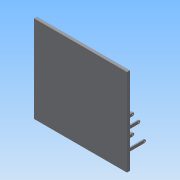
# Autodesk Inventor part: 0
Saved by Autodesk Inventor 2015 (Build 190159000, 159)
## iProperties
Created: 2018-05-07
Part Number: 0
Material: 一般
Document SubType Name: Modeling
Designer: 王博聖
Density: 1 g/cm^3
Appearance: 預設
Author: 王博聖
Autodesk Inventor part; units mm, degrees
ref_plane "YZ Plane" through (0, 0, 0) normal (1, 0, 0) x (0, 1, 0)
ref_plane "XZ Plane" through (0, 0, 0) normal (0, 1, 0) x (-1, 0, 0)
sketch "草圖1" plane through (0, 0, 0) normal (0, 1, 0) x (-1, 0, 0)
  line L0 (0, 0) -> (160, 0)
  line L1 (160, 0) -> (160, -130)
  line L2 (160, -130) -> (0, -130)
  line L3 (0, -130) -> (0, 0)
  dimension "d0" = 160
  dimension "d1" = 130
  constraints: 8 end point, 2 parallel, 1 horizontal, 1 perpendicular
  measures "d0" distance of L1.end L2.end
  measures "d1" distance of L0.end L1.end
extrude "擠出1" add sketch "草圖1" along normal blind 5
sketch "草圖2" plane through (0, 0, 0) normal (1, 0, 0) x (0, 0, -1)
  line L0 (130, 0) -> (0, 0) projected
  line L1 (65, 0) -> (65, 20.4)
  line L2 (65, 20.4) -> (65, 0) construction
  line L3 (62.5, 20.4) -> (62.5, 0)
  line L4 (67.5, 0) -> (67.5, 20.4)
  arc A0 (67.5, 20.4) -> (62.5, 20.4) centre (65, 20.4) ccw
  arc A1 (62.5, 0) -> (67.5, 0) centre (65, 0) ccw construction
  line L5 (67.5, 0) -> (62.5, 0)
  circle A2 centre (65, 20.4) radius 1.25
  point P0 (65, 10.2)
  dimension "d4" = 20.4
  dimension "d5" = 5
  dimension "d6" = 2.5
  constraints: 12 end point, 4 point on circle, 4 tangent, 3 centre point, 2 collinear, 2 midpoint, 1 coincident, 1 parallel, 1 vertical
  measures "d4" distance of L1.start L1.end
  measures "d5" diameter of A1
  measures "d6" diameter of A2
extrude "擠出2" add sketch "草圖2" against normal blind 2
sketch "草圖3" plane through (0, 0, 0) normal (1, 0, 0) x (0, 0, -1)
  line L0 (130, 0) -> (0, 0) construction
  arc A0 (67.5, 20.4) -> (62.5, 20.4) centre (65, 20.4) ccw projected
  line L1 (65, 20.4) -> (48.2, 20.4) construction
  line L2 (48.2, 20.4) -> (48.2, 10) construction
  line L3 (48.2, 10) -> (48.2, 0) construction
  line L4 (45.7, 10) -> (45.7, 0)
  line L5 (50.7, 0) -> (50.7, 10)
  arc A1 (50.7, 10) -> (45.7, 10) centre (48.2, 10) ccw
  arc A2 (45.7, 0) -> (50.7, 0) centre (48.2, 0) ccw construction
  circle A3 centre (48.2, 10) radius 1.25
  line L6 (50.7, 0) -> (45.7, 0)
  line L7 (65, 20.4) -> (42, 20.4) construction
  line L8 (42, 20.4) -> (42, 10) construction
  line L9 (42, 10) -> (42, 0) construction
  line L10 (39.5, 10) -> (39.5, 0)
  line L11 (44.5, 0) -> (44.5, 10)
  arc A4 (44.5, 10) -> (39.5, 10) centre (42, 10) ccw
  arc A5 (39.5, 0) -> (44.5, 0) centre (42, 0) ccw construction
  circle A6 centre (42, 10) radius 1.25
  line L12 (44.5, 0) -> (39.5, 0)
  circle A7 centre (65, 20.4) radius 1.25 projected
  line L13 (65, 20.4) -> (78.6, 20.4) construction
  line L14 (78.6, 20.4) -> (78.6, 10) construction
  line L15 (78.6, 10) -> (78.6, 0) construction
  line L16 (76.1, 10) -> (76.1, 0)
  line L17 (81.1, 0) -> (81.1, 10)
  arc A8 (81.1, 10) -> (76.1, 10) centre (78.6, 10) ccw
  arc A9 (76.1, 0) -> (81.1, 0) centre (78.6, 0) ccw construction
  circle A10 centre (78.6, 10) radius 1.25
  line L18 (81.1, 0) -> (76.1, 0)
  line L19 (81.1, 0) -> (76.1, 0)
  line L20 (0, 0) -> (130, 0) projected
  line L21 (65, 20.4) -> (65, 30.17) construction
  line L22 (65, 30.17) -> (98.58, 30.17) construction
  line L23 (98.58, 30.17) -> (98.58, 0) construction
  line L24 (96.08, 30.17) -> (96.08, 0)
  line L25 (101.08, 0) -> (101.08, 30.17)
  arc A11 (101.08, 30.17) -> (96.08, 30.17) centre (98.58, 30.17) ccw
  arc A12 (96.08, 0) -> (101.08, 0) centre (98.58, 0) ccw construction
  circle A13 centre (98.58, 30.17) radius 1.25
  line L26 (101.08, 0) -> (96.08, 0)
  point P0 (48.2, 5)
  point P1 (42, 5)
  point P2 (78.6, 5)
  point P3 (98.58, 15.085)
  dimension "d9" = 16.8
  dimension "d11" = 10.4
  dimension "d12" = 5
  dimension "d13" = 2.5
  dimension "d14" = 23
  dimension "d15" = 10.4
  dimension "d16" = 5
  dimension "d17" = 2.5
  dimension "d20" = 13.6
  dimension "d21" = 10.4
  dimension "d22" = 5
  dimension "d23" = 2.5
  dimension "d24" = 9.77
  dimension "d25" = 33.58
  dimension "d26" = 5
  dimension "d27" = 2.5
  constraints: 58 end point, 16 point on circle, 16 tangent, 12 centre point, 8 perpendicular, 4 coincident, 4 horizontal, 4 midpoint, 4 parallel, 4 point on line, 3 collinear, 2 vertical
  measures "d9" distance of L1.start L1.end
  measures "d11" distance of L1.end L2.end
  measures "d12" diameter of A2
  measures "d13" diameter of A3
  measures "d14" distance of L1.start L7.end
  measures "d15" distance of L7.end L8.end
  measures "d16" diameter of A5
  measures "d17" diameter of A6
  measures "d20" distance of L13.start L13.end
  measures "d21" distance of L13.end L14.end
  measures "d22" diameter of A9
  measures "d23" diameter of A10
  measures "d24" distance of L13.start L21.end
  measures "d25" distance of L21.end L22.end
  measures "d26" diameter of A12
  measures "d27" diameter of A13
extrude "擠出3" add sketch "草圖3" against normal blind 2 contours A1 L5 L6 L4 | L24 A11 L25 L20 | L16 A8 L17 L18 | L12 L10 A4 L11
sketch "草圖4" plane through (-160, 0, 0) normal (0, 0, 1) x (1, 0, 0)
  line L0 (160, 0) -> (0, 0) projected
  line L1 (160, 0) -> (160, 5) projected
  line L2 (0, 5) -> (160, 5) projected
  line L3 (0, 0) -> (0, 5) projected
extrude "擠出4" add sketch "草圖4" along normal blind 20
sketch "草圖5" plane through (-2, 0, 0) normal (-1, 0, 0) x (0, 0, 1)
  line L0 (-45.7, 5) -> (-50.7, 5) projected
  line L1 (-45.7, 5) -> (-45.7, 10) projected
  arc A0 (-45.7, 10) -> (-50.7, 10) centre (-48.2, 10) ccw projected
  line L2 (-50.7, 10) -> (-50.7, 5) projected
  circle A1 centre (-48.2, 10) radius 1.25 projected
  line L3 (-76.1, 5) -> (-81.1, 5) projected
  line L4 (-76.1, 5) -> (-76.1, 10) projected
  arc A2 (-76.1, 10) -> (-81.1, 10) centre (-78.6, 10) ccw projected
  line L5 (-81.1, 10) -> (-81.1, 5) projected
  circle A3 centre (-78.6, 10) radius 1.25 projected
  point P0 (0, 0)
extrude "擠出5" add sketch "草圖5" along normal blind 2
ref_plane "工作平面1" through (-12, 0, -130) normal (1, 0, 0) x (0, 0, -1)
sketch "草圖6" plane through (-12, 0, -130) normal (1, 0, 0) x (0, 0, -1)
  line L0 (-90.5, 5) -> (-85.5, 5) projected
  line L1 (-90.5, 5) -> (-90.5, 10) projected
  arc A0 (-85.5, 10) -> (-90.5, 10) centre (-88, 10) ccw projected
  line L2 (-85.5, 10) -> (-85.5, 5) projected
  circle A1 centre (-88, 10) radius 1.25 projected
  point P0 (-130, 0)
extrude "擠出6" add sketch "草圖6" against normal blind 2
extrude "擠出7" cut sketch "草圖6" along normal blind 20
